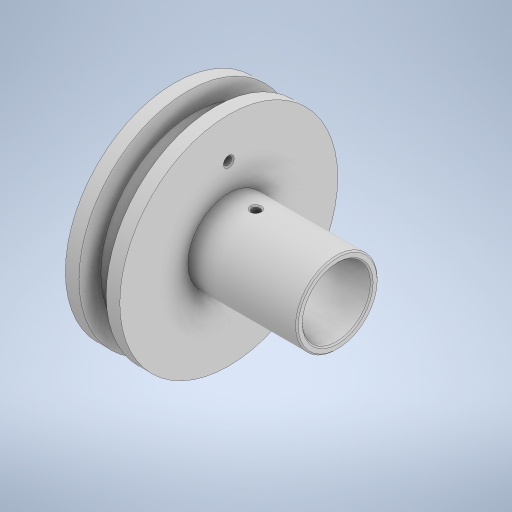
# Autodesk Inventor part: Шкив 80
Saved by Autodesk Inventor 2023 (Build 270158000, 158)
## iProperties
Created: 2022-05-01
Part Number: Шкив 80
Material: Типовые
Document SubType Name: Modeling
Designer: User
Density: 1 g/cm^3
Appearance: По умолчанию
Author: User
Autodesk Inventor part; units mm, degrees
ref_plane "YZ Plane" through (0, 0, 0) normal (1, 0, 0) x (0, 1, 0)
sketch "Эскиз1" plane through (0, 0, 0) normal (0, 1, 0) x (-1, 0, 0)
  line L0 (0, 0) -> (20, 0)
  line L1 (20, 0) -> (20, 40)
  line L2 (20, 40) -> (0, 40)
  line L3 (0, 40) -> (0, 0)
  line L4 (20, 40) -> (13, 40)
  line L5 (13, 40) -> (13, 34)
  line L6 (13, 34) -> (7, 34)
  line L7 (7, 34) -> (7, 40)
  dimension "d0" = 20
  dimension "d1" = 40
  dimension "d2" = 7
  dimension "d3" = 6
  dimension "d4" = 6
  constraints: 16 end point, 6 perpendicular, 2 point on line, 1 horizontal
  measures "d0" distance of L0.start L0.end
  measures "d1" distance of L0.end L1.end
  measures "d2" distance of L1.end L4.end
  measures "d3" distance of L4.end L5.end
  measures "d4" distance of L5.end L6.end
revolve "Вращение1" add sketch "Эскиз1" angle 360 about axis through (0, 0, 0) along (-1, 0, 0) contours L3 L2 L7 L6 L5 L1 L0
sketch "Эскиз2" plane through (0, 0, 0) normal (1, 0, 0) x (0, 0, -1)
  circle A0 centre (0, 0) radius 15
  dimension "d6" = 30
  constraints: 1 centre point, 1 coincident
  measures "d6" diameter of A0
extrude "Выдавливание1" add sketch "Эскиз2" along normal blind 40
sketch "Эскиз3" plane through (40, 0, 0) normal (1, 0, 0) x (0, 0, -1)
  circle A0 centre (0, 0) radius 12.5
  dimension "d9" = 25
  constraints: 1 centre point, 1 coincident
  measures "d9" diameter of A0
extrude "Выдавливание2" cut sketch "Эскиз3" against normal blind 88.25
chamfer "Фаска1" distance 2 distance2 6 1 edges at (-13, 0, -40) measured on face at (-17.6667, 18.0952, -35.673)
chamfer "Фаска2" distance 6 distance2 2 1 edges at (-7, 0, -40) measured on face at (-7, -32.7494, -18.8557)
sketch "Эскиз4" plane through (0, 0, 0) normal (1, 0, 0) x (0, 0, -1)
  circle A0 centre (0, 0) radius 15 projected
  point P0 (0, 15)
  constraints: 1 vertical alignment, 1 other
ref_plane "РабПлоскость1" through (0, 15, 0) normal (0, 1, 0) x (-1, 0, 0)
sketch "Эскиз5" plane through (0, 15, 0) normal (0, 1, 0) x (-1, 0, 0)
  line L0 (0, 0) -> (-10, 0)
  circle A0 centre (-10, 0) radius 1.5
  dimension "d18" = 10
  dimension "d19" = 3
  constraints: 2 end point, 1 centre point, 1 coincident, 1 horizontal
  measures "d18" distance of L0.start L0.end
  measures "d19" diameter of A0
extrude "Выдавливание3" cut sketch "Эскиз5" against normal blind 58
thread "Резьба1" size "M3x0.5" class "6H" standard "ISO Metric profile" full length
chamfer "Фаска3" distance 0.5 angle 45 5 edges at (11.4169, -14.9919, 0.4923) (10.1368, 14.9254, -1.4937) (9.9997, 14.9248, 1.5) (40, 0, 15) (40, 0, 12.5)
ref_plane "РабПлоскость2" through (-10, 0, 0) normal (-1, 0, 0) x (0, 0, 1)
sketch "Эскиз6" plane through (0, 0, 0) normal (1, 0, 0) x (0, 0, -1)
  circle A0 centre (0, 0) radius 15 projected
  line L0 (0, 0) -> (0, 25)
  circle A1 centre (0, 25) radius 1.5
  dimension "d28" = 25
  dimension "d29" = 3
  constraints: 2 end point, 1 centre point, 1 coincident, 1 vertical
  measures "d28" distance of L0.start L0.end
  measures "d29" diameter of A1
extrude "Выдавливание4" cut sketch "Эскиз6" against normal blind 59.75 contours A1
chamfer "Фаска4" distance 0.5 angle 45 1 edges at (0, 25, 1.5)
chamfer "Фаска5" distance 0.5 angle 45 1 edges at (-20, 25, 1.5)
